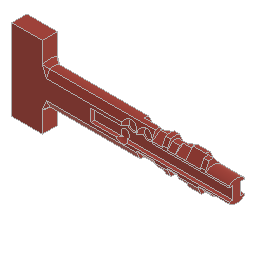
Protec (cam compatible) (Autodesk Fusion 360 design; units mm, degrees)
Autodesk Fusion 360 part; units mm, degrees
note: some values were not read from the file. Chosen so that the rebuilt part matches the saved one: which pieces of a blend or face edit are solid.
sketch "profile" plane through (0, 0, 0) normal (1, 0, 0) x (0, 1, 0)
  line L0 (0, 0) -> (3.3, 0) construction
  line L1 (3.3, 0) -> (3.3, 3.3) construction
  line L2 (3.3, 3.3) -> (4.05, 3.3) construction
  line L3 (3.3, 3.3) -> (2.55, 3.3) construction
  line L4 (4.05, 3.3) -> (4.05, 4.5)
  line L5 (4.05, 3.3) -> (4.05, 2.1)
  line L6 (2.55, 3.3) -> (2.55, 4.5)
  line L7 (2.55, 3.3) -> (2.55, 2.1)
  line L8 (4.05, 4.5) -> (4.775, 4.5)
  line L9 (4.05, 2.1) -> (4.775, 2.1)
  line L10 (2.55, 2.1) -> (1.825, 2.1)
  line L11 (2.55, 4.5) -> (1.825, 4.5)
  line L12 (4.775, 4.5) -> (4.775, 5.165)
  line L13 (4.775, 2.1) -> (4.775, 1.435)
  line L14 (1.825, 2.1) -> (1.825, 1.435)
  line L15 (1.825, 4.5) -> (1.825, 5.165)
  line L16 (4.775, 5.165) -> (4.1589, 6.4863)
  line L17 (4.775, 5.165) -> (1.825, 5.165) construction
  line L18 (1.825, 1.435) -> (2.4411, 0.1137)
  line L19 (1.825, 5.165) -> (2.4411, 6.4863)
  line L20 (1.825, 5.165) -> (4.775, 5.165) construction
  line L21 (4.775, 1.435) -> (4.1589, 0.1137)
  arc A0 (4.1589, 6.4863) -> (2.4411, 6.4863) centre (3.3, 3.3) ccw
  arc A1 (2.4411, 0.1137) -> (4.1589, 0.1137) centre (3.3, 3.3) ccw
  dimension "d1" = 3.3
  dimension "d2" = 3.3
  dimension "d3" = 0.75
  dimension "d4" = 1.2
  dimension "d5" = 0.725
  dimension "d6" = 65
  dimension "d7" = 65
  dimension "d8" = 3.3
  dimension "d9" = 4.25
  constraint coincident L0.start origin
  constraint horizontal L0
  constraint perpendicular L0 L1
  constraint perpendicular L1 L2
  constraint perpendicular L1 L3
  constraint equal L2 L3
  constraint perpendicular L2 L4
  constraint perpendicular L2 L5
  constraint perpendicular L3 L6
  constraint perpendicular L3 L7
  constraint perpendicular L4 L8
  constraint perpendicular L5 L9
  constraint perpendicular L7 L10
  constraint perpendicular L6 L11
  constraint equal L6 L7
  constraint equal L5 L7
  constraint equal L4 L5
  constraint equal L8 L9
  constraint equal L9 L10
  constraint equal L10 L11
  constraint perpendicular L8 L12
  constraint perpendicular L9 L13
  constraint perpendicular L10 L14
  constraint perpendicular L11 L15
  constraint equal L12 L15
  constraint equal L14 L15
  constraint equal L13 L14
  constraint horizontal L17
  constraint parallel L16 L18
  constraint horizontal L20
  constraint equal L16 L19
  constraint parallel L19 L21
  constraint equal L18 L21
  constraint equal L16 L18
  constraint coincident L1.end L2.start
  measures "d1" distance of L0.start L0.end
  measures "d2" distance of L0.end L1.end
  measures "d3" distance of L1.end L2.end
  measures "d4" distance of L2.end L4.end
  measures "d5" distance of L4.end L8.end
  measures "d6" angle of L16 L17
  measures "d7" angle of L19 L20
  measures "d8" radius of A0
  measures "d9" distance of L16 L18
extrude "Extrude1" add sketch "profile" against normal blind 42.57 makes body 1
ref_plane "WorkPlane1" through (-21.285, 3.3, 3.3) normal (0, -1, 0) x (0, 0, 1)
sketch "bow" plane through (-42.57, 0, 0) normal (-1, 0, 0) x (0, -1, 0)
  line L0 (-2.55, 2.1) -> (-2.55, 4.5)
  line L1 (-2.55, 4.5) -> (-1.825, 4.5)
  line L2 (-1.825, 4.5) -> (-1.825, 5.165)
  line L3 (-1.825, 5.165) -> (-2.4411, 6.4863)
  arc A0 (-2.4411, 6.4863) -> (-4.1589, 6.4863) centre (-3.3, 3.3) ccw
  line L4 (-4.1589, 6.4863) -> (-4.775, 5.165)
  line L5 (-4.775, 5.165) -> (-4.775, 4.5)
  line L6 (-4.775, 4.5) -> (-4.05, 4.5)
  line L7 (-4.05, 4.5) -> (-4.05, 2.1)
  line L8 (-4.05, 2.1) -> (-4.775, 2.1)
  line L9 (-4.775, 2.1) -> (-4.775, 1.435)
  line L10 (-4.775, 1.435) -> (-4.1589, 0.1137)
  arc A1 (-4.1589, 0.1137) -> (-2.4411, 0.1137) centre (-3.3, 3.3) ccw
  line L11 (-2.4411, 0.1137) -> (-1.825, 1.435)
  line L12 (-1.825, 1.435) -> (-1.825, 2.1)
  line L13 (-1.825, 2.1) -> (-2.55, 2.1)
  circle A2 centre (-3.3, 3.3) radius 3.3 construction
  line L14 (-1.825, 5.165) -> (-1.825, 6.252)
  line L15 (-4.775, 5.165) -> (-4.775, 6.252)
  line L16 (-1.825, 1.435) -> (-1.825, 0.348)
  line L17 (-4.775, 1.435) -> (-4.775, 0.348)
  line L18 (-1.825, 6.252) -> (-1.825, 11.252)
  line L19 (-4.775, 6.252) -> (-4.775, 11.252)
  line L20 (-1.825, 0.348) -> (-1.825, -4.652)
  line L21 (-4.775, 0.348) -> (-4.775, -4.652)
  line L22 (-1.825, 11.252) -> (-4.775, 11.252)
  line L23 (-4.775, -4.652) -> (-1.825, -4.652)
  line L24 (-1.825, 1.435) -> (-1.825, 5.165)
  line L25 (-4.775, 5.165) -> (-4.775, 1.435)
  point P0 (-1.825, 5.165)
  point P1 (-4.775, 5.165)
  point P2 (-4.775, 1.435)
  point P3 (-1.825, 1.435)
  dimension "d12" = 6.6
  dimension "d13" = 5
  constraint concentric A0 A2
  constraint coincident P0 L2.end
  constraint coincident A2 L14.end
  constraint parallel L2 L14
  constraint coincident P1 L4.end
  constraint coincident A2 L15.end
  constraint parallel L5 L15
  constraint coincident P3 L11.end
  constraint coincident A2 L16.end
  constraint parallel L12 L16
  constraint coincident P2 L9.end
  constraint coincident A2 L17.end
  constraint parallel L9 L17
  constraint parallel L14 L18
  constraint parallel L15 L19
  constraint parallel L16 L20
  constraint parallel L17 L21
  constraint equal L20 L21
  constraint equal L19 L21
  constraint equal L18 L19
  measures "d12" diameter of A2
  measures "d13" distance of L14.end L18.end
sketch "dss holes + dc align" plane through (0, 3.3, 0) normal (0, -1, 0) x (-1, 0, 0)
  line L0 (0, 0) -> (0, -3.3) construction
  line L1 (0, -3.3) -> (19.57, -3.3) construction
  line L2 (19.57, -3.3) -> (21.07, -3.3) construction
  line L3 (21.07, -3.3) -> (21.07, -4.1) construction
  line L4 (21.07, -3.3) -> (21.07, -2.5) construction
  line L5 (19.57, -3.3) -> (19.57, -4.9) construction
  line L6 (19.57, -3.3) -> (19.57, -1.7) construction
  circle A0 centre (19.57, -4.9) radius 0.9
  circle A1 centre (19.57, -1.7) radius 0.9
  circle A2 centre (16.57, -4.9) radius 0.9
  circle A3 centre (16.57, -1.7) radius 0.9
  point P0 (21.07, -4.1)
  point P1 (21.07, -2.5)
  dimension "d14" = 3.3
  dimension "d15" = 19.57
  dimension "d16" = 1.5
  dimension "d17" = 0.8
  dimension "d18" = 1.6
  dimension "d19" = 1.8
  dimension "d20" = 3
  dimension "d21" = 1.6
  dimension "d22" = 3
  dimension "d23" = 1.6
  constraint coincident L0.start origin
  constraint vertical L0
  constraint perpendicular L0 L1
  constraint parallel L1 L2
  constraint perpendicular L2 L3
  constraint perpendicular L2 L4
  constraint equal L3 L4
  constraint perpendicular L2 L5
  constraint perpendicular L2 L6
  constraint equal L5 L6
  constraint coincident L5.end A0.centre
  constraint coincident L6.end A1.centre
  constraint equal A0 A1
  constraint equal A0 A2
  constraint equal A0 A3
  constraint coincident P0 L3.end
  constraint coincident P1 L4.end
  measures "d14" distance of L0.start L0.end
  measures "d15" distance of L0.end L1.end
  measures "d16" distance of L1.end L2.end
  measures "d17" distance of L2.end P0
  measures "d18" distance of L1.end L5.end
  measures "d19" diameter of A0
  measures "d20" distance of L5.end A2.centre
  measures "d21" distance of L1 A2.centre
  measures "d22" distance of L6.end A3.centre
  measures "d23" distance of L1 A3.centre
sketch "dc bearings" plane through (0, 0, 0) normal (1, 0, 0) x (0, 1, 0)
  line L0 (0, 0) -> (3.3, 0) construction
  line L1 (3.3, 0) -> (3.3, 3.3) construction
  line L2 (3.3, 3.3) -> (1.4542, 2.8398) construction
  line L3 (3.3, 3.3) -> (2.3, 3.3) construction
  line L4 (3.3, 3.3) -> (5.1458, 3.7602) construction
  circle A0 centre (1.4542, 2.8398) radius 1.375
  circle A1 centre (5.1458, 3.7602) radius 1.375
  point P0 (1.4542, 2.8398)
  point P1 (5.1458, 3.7602)
  dimension "d24" = 3.3
  dimension "d25" = 3.3
  dimension "d26" = 14
  dimension "d27" = 1.9023
  dimension "d28" = 1
  dimension "d29" = 2.75
  constraint coincident L0.start origin
  constraint horizontal L0
  constraint perpendicular L0 L1
  constraint horizontal L3
  constraint parallel L2 L4
  constraint equal L2 L4
  constraint coincident P0 L2.end
  constraint coincident P1 L4.end
  constraint equal A0 A1
  measures "d24" distance of L0.start L0.end
  measures "d25" distance of L0.end L1.end
  measures "d26" angle of L2 L3
  measures "d27" distance of L1.end P0
  measures "d28" distance of L1.end L3.end
  measures "d29" diameter of A0
extrude "bow (1)" add sketch "bow" against normal blind 6 bodies 1
extrude "shaft strength" add 2 faces at (-36.57, 2.3083, 2.9) (-36.57, 4.5333, 3.7) along direction (1, 0, 0) blind 9.5 on bodies 1 bodies 1
chamfer "Chamfer1" distance 0.8 angle 45 6 edges at (-36.57, 2.1331, 5.8256) (-36.57, 3.3, 6.6) (-36.57, 2.1331, 0.7744) (-36.57, 4.4669, 5.8256) (-36.57, 3.3, 0) (-36.57, 4.4669, 0.7744) on bodies 1
extrude "dc bearings (1)" add sketch "dc bearings" along normal mid plane 2.75 separate body makes body 2 at (0.9167, 6.5191, 3.6917) makes body 3 at (0.9167, 2.8275, 2.7712)
fillet "Fillet1" radius 1.375 4 edges at (-1.375, 3.8639, 4.2574) (1.375, 3.8639, 3.263) (-1.375, 0.1722, 3.337) (1.375, 0.1722, 2.3426) on bodies 2 3
move_body "Move1" bodies 2 3 to x (1, 0, 0) y (0, 1, 0) z (0, 0, 1) at (-21.07, 0, 0)
extrude "Extrude5" cut sketch "dss holes + dc align" along normal blind 0.9 draft 35 from surface at 0.575 contours A0 | A2 bodies 1
extrude "Extrude6" cut sketch "dss holes + dc align" against normal blind 0.9 draft 35 from surface at -0.575 contours A1 | A3 bodies 1
combine "Combine1" operation cut target body 1 tool bodies 2 3
sketch "1 cut" plane through (0, 0, 0) normal (1, 0, 0) x (0, 1, 0)
  line L0 (0, 0) -> (3.3, 0) construction
  line L1 (3.3, 0) -> (3.3, 3.3) construction
  line L2 (3.3, 3.3) -> (4.05, 3.3) construction
  line L3 (4.05, 3.3) -> (4.05, 4.5)
  line L4 (4.05, 4.5) -> (4.775, 4.5)
  line L5 (4.05, 3.3) -> (4.05, 2.1)
  line L6 (4.05, 2.1) -> (4.775, 2.1)
  line L7 (2.55, 2.1) -> (1.825, 2.1)
  line L8 (2.55, 3.3) -> (2.55, 2.1)
  line L9 (2.55, 3.3) -> (2.55, 4.5)
  line L10 (2.55, 4.5) -> (1.825, 4.5)
  line L11 (4.775, 4.5) -> (4.775, 4.8481)
  line L12 (1.825, 2.1) -> (1.825, 1.7519)
  line L13 (1.825, 4.5) -> (1.825, 5.165)
  line L14 (4.775, 2.1) -> (4.775, 1.435)
  circle A0 centre (3.3, 3.3) radius 3.3 construction
  line L15 (4.775, 4.8481) -> (3.305, 6.6)
  line L16 (4.775, 4.8481) -> (1.825, 4.8481) construction
  line L17 (1.825, 1.7519) -> (3.295, 0)
  line L18 (1.825, 5.165) -> (2.4411, 6.4863)
  line L19 (1.825, 5.165) -> (4.509, 5.165) construction
  line L20 (4.775, 1.435) -> (4.1589, 0.1137)
  arc A1 (3.305, 6.6) -> (2.4411, 6.4863) centre (3.3, 3.3) ccw
  arc A2 (3.295, 0) -> (4.1589, 0.1137) centre (3.3, 3.3) ccw
  circle A3 centre (3.3, 3.3) radius 4.125
  dimension "d48" = 3.3
  dimension "d49" = 3.3
  dimension "d50" = 0.75
  dimension "d51" = 1.2
  dimension "d52" = 0.725
  dimension "d53" = 6.6
  dimension "d54" = 50
  dimension "d55" = 4.25
  dimension "d56" = 65
  dimension "d57" = 4.25
  dimension "d58" = 3.3
  dimension "d59" = 3.3
  dimension "d60" = 8.25
  constraint coincident L0.start origin
  constraint horizontal L0
  constraint perpendicular L0 L1
  constraint perpendicular L1 L2
  constraint perpendicular L2 L3
  constraint perpendicular L3 L4
  constraint perpendicular L2 L5
  constraint perpendicular L5 L6
  constraint equal L3 L5
  constraint equal L4 L6
  constraint symmetric L1 L2.end L8.start
  constraint symmetric L1 L3.end L9.end
  constraint symmetric L1 L4.end L10.end
  constraint symmetric L1 L5.end L7.start
  constraint symmetric L1 L6.end L7.end
  constraint perpendicular L4 L11
  constraint perpendicular L7 L12
  constraint equal L11 L12
  constraint perpendicular L10 L13
  constraint perpendicular L6 L14
  constraint equal L13 L14
  constraint coincident L1.end L2.start
  constraint horizontal L16
  constraint coincident A0 L15.end
  constraint coincident A0 L17.end
  constraint parallel L15 L17
  constraint horizontal L19
  constraint coincident A0 L18.end
  constraint coincident A0 L20.end
  constraint parallel L18 L20
  constraint coincident L13 L16.end
  constraint coincident L15 L19.end
  constraint concentric A2 A3
  measures "d48" distance of L0.start L0.end
  measures "d49" distance of L0.end L1.end
  measures "d50" distance of L1.end L2.end
  measures "d51" distance of L2.end L3.end
  measures "d52" distance of L3.end L4.end
  measures "d53" diameter of A0
  measures "d54" angle of L15 L16
  measures "d55" distance of L15 L17
  measures "d56" angle of L18 L19
  measures "d57" distance of L18 L20
  measures "d58" radius of A1
  measures "d59" radius of A2
  measures "d60" diameter of A3
sketch "2 cut" plane through (0, 0, 0) normal (1, 0, 0) x (0, 1, 0)
  line L0 (1.825, 5.165) -> (2.4411, 6.4863) construction
  line L1 (1.825, 4.5) -> (1.825, 5.165) construction
  line L2 (2.55, 4.5) -> (1.825, 4.5) construction
  line L3 (2.55, 3.3) -> (2.55, 4.5) construction
  line L4 (2.55, 3.3) -> (2.55, 2.1) construction
  line L5 (2.55, 2.1) -> (1.825, 2.1) construction
  line L6 (1.825, 2.1) -> (1.825, 1.7519) construction
  line L7 (1.825, 1.7519) -> (3.295, 0) construction
  arc A0 (3.295, 0) -> (4.1589, 0.1137) centre (3.3, 3.3) ccw construction
  line L8 (4.775, 1.435) -> (4.1589, 0.1137) construction
  line L9 (4.775, 2.1) -> (4.775, 1.435) construction
  line L10 (4.05, 2.1) -> (4.775, 2.1) construction
  line L11 (4.05, 3.3) -> (4.05, 2.1) construction
  line L12 (4.05, 3.3) -> (4.05, 4.5) construction
  line L13 (4.05, 4.5) -> (4.775, 4.5) construction
  line L14 (4.775, 4.5) -> (4.775, 4.8481) construction
  arc A1 (3.305, 6.6) -> (2.4411, 6.4863) centre (3.3, 3.3) ccw construction
  line L15 (4.775, 4.8481) -> (3.305, 6.6) construction
  circle A2 centre (3.3, 3.3) radius 4.125 construction
  line L16 (3.3, 3.3) -> (3.3, 4.3) construction
  line L17 (4.775, 5.165) -> (4.1589, 6.4863)
  line L18 (4.775, 4.5) -> (4.775, 5.165)
  line L19 (4.05, 4.5) -> (4.775, 4.5)
  line L20 (4.05, 3.3) -> (4.05, 4.5)
  line L21 (4.05, 3.3) -> (4.05, 2.1)
  line L22 (4.05, 2.1) -> (4.775, 2.1)
  line L23 (4.775, 2.1) -> (4.775, 1.7519)
  line L24 (4.775, 1.7519) -> (3.305, 0)
  arc A3 (2.4411, 0.1137) -> (3.305, 0) centre (3.3, 3.3) ccw
  line L25 (1.825, 1.435) -> (2.4411, 0.1137)
  line L26 (1.825, 2.1) -> (1.825, 1.435)
  line L27 (2.55, 2.1) -> (1.825, 2.1)
  line L28 (2.55, 3.3) -> (2.55, 2.1)
  line L29 (2.55, 3.3) -> (2.55, 4.5)
  line L30 (2.55, 4.5) -> (1.825, 4.5)
  line L31 (1.825, 4.5) -> (1.825, 4.8481)
  arc A4 (4.1589, 6.4863) -> (3.295, 6.6) centre (3.3, 3.3) ccw
  line L32 (1.825, 4.8481) -> (3.295, 6.6)
  circle A5 centre (3.3, 3.3) radius 4.125
  dimension "d61" = 1
  constraint coincident A0.centre A1.centre
  constraint parallel L3 L16
  constraint symmetric L0.start L16 L17.start
  constraint symmetric L0.end L16 L17.end
  constraint symmetric L1.start L16 L13.end
  constraint symmetric L2.start L16 L12.end
  constraint symmetric L3.start L16 L11.start
  constraint symmetric L4.end L16 L10.start
  constraint symmetric L5.end L16 L9.start
  constraint symmetric L6.end L16 L23.end
  constraint symmetric L7.end L16 L24.end
  constraint symmetric A0.end L16 A3.start
  constraint symmetric A0 L16 A3
  constraint symmetric L8.start L16 L25.start
  constraint symmetric L9.start L16 L5.end
  constraint symmetric L10.start L16 L4.end
  constraint symmetric L11.start L16 L3.start
  constraint symmetric L12.end L16 L2.start
  constraint symmetric L13.end L16 L1.start
  constraint symmetric L14.end L16 L31.end
  constraint symmetric A1.start L16 A4.end
  constraint symmetric A1 L16 A4
  constraint symmetric A2 L16 A5
  measures "d61" distance of A0.centre L16.end
sketch "3 cut" plane through (0, 0, 0) normal (1, 0, 0) x (0, 1, 0)
  line L0 (0, 0) -> (3.3, 0) construction
  line L1 (3.3, 0) -> (3.3, 3.3) construction
  line L2 (3.3, 3.3) -> (4.05, 3.3) construction
  line L3 (2.55, 3.3) -> (2.55, 2.1)
  line L4 (2.55, 2.1) -> (1.825, 2.1)
  line L5 (2.55, 3.3) -> (2.55, 4.5)
  line L6 (2.55, 4.5) -> (1.825, 4.5)
  line L7 (4.05, 4.5) -> (4.775, 4.5)
  line L8 (4.05, 3.3) -> (4.05, 4.5)
  line L9 (4.05, 3.3) -> (4.05, 2.1)
  line L10 (4.05, 2.1) -> (4.775, 2.1)
  line L11 (4.775, 4.5) -> (4.775, 4.8613)
  line L12 (1.825, 2.1) -> (1.825, 1.7387)
  line L13 (1.825, 4.5) -> (1.825, 5.165)
  line L14 (4.775, 2.1) -> (4.775, 1.435)
  circle A0 centre (3.3, 3.3) radius 2.7 construction
  line L15 (4.775, 4.8613) -> (3.1544, 5.9961)
  line L16 (4.775, 4.8613) -> (1.825, 4.8613) construction
  line L17 (1.825, 1.7387) -> (3.4456, 0.6039)
  line L18 (1.825, 5.165) -> (2.078, 5.7077)
  line L19 (1.825, 5.165) -> (4.3413, 5.165) construction
  line L20 (4.775, 1.435) -> (4.522, 0.8923)
  arc A1 (3.1544, 5.9961) -> (2.078, 5.7077) centre (3.3, 3.3) ccw
  arc A2 (3.4456, 0.6039) -> (4.522, 0.8923) centre (3.3, 3.3) ccw
  circle A3 centre (3.3, 3.3) radius 4.125
  dimension "d62" = 3.3
  dimension "d63" = 3.3
  dimension "d64" = 0.75
  dimension "d65" = 5.4
  dimension "d66" = 35
  dimension "d67" = 4.25
  dimension "d68" = 65
  dimension "d69" = 4.25
  dimension "d70" = 2.7
  dimension "d71" = 2.7
  dimension "d72" = 8.25
  constraint coincident L0.start origin
  constraint horizontal L0
  constraint perpendicular L0 L1
  constraint perpendicular L1 L2
  constraint coincident L7.end L11.start
  constraint perpendicular L7 L11
  constraint coincident L4.end L12.start
  constraint perpendicular L4 L12
  constraint equal L11 L12
  constraint coincident L6.end L13.start
  constraint perpendicular L6 L13
  constraint coincident L10.end L14.start
  constraint perpendicular L10 L14
  constraint equal L13 L14
  constraint coincident L1.end L2.start
  constraint horizontal L16
  constraint coincident A0 L15.end
  constraint coincident A0 L17.end
  constraint parallel L15 L17
  constraint horizontal L19
  constraint coincident A0 L18.end
  constraint coincident A0 L20.end
  constraint parallel L18 L20
  constraint concentric A2 A3
  constraint coincident L13 L16.end
  constraint coincident L15 L19.end
  measures "d62" distance of L0.start L0.end
  measures "d63" distance of L0.end L1.end
  measures "d64" distance of L1.end L2.end
  measures "d65" diameter of A0
  measures "d66" angle of L15 L16
  measures "d67" distance of L15 L17
  measures "d68" angle of L18 L19
  measures "d69" distance of L18 L20
  measures "d70" radius of A2
  measures "d71" radius of A1
  measures "d72" diameter of A3
sketch "4 cut" plane through (0, 0, 0) normal (1, 0, 0) x (0, 1, 0)
  line L0 (0, 0) -> (3.3, 0) construction
  line L1 (3.3, 0) -> (3.3, 3.3) construction
  line L2 (3.3, 3.3) -> (4.05, 3.3) construction
  line L3 (2.55, 4.5) -> (1.825, 4.5)
  line L4 (2.55, 3.3) -> (2.55, 4.5)
  line L5 (2.55, 3.3) -> (2.55, 2.1)
  line L6 (2.55, 2.1) -> (1.825, 2.1)
  line L7 (4.05, 2.1) -> (4.775, 2.1)
  line L8 (4.05, 3.3) -> (4.05, 2.1)
  line L9 (4.05, 3.3) -> (4.05, 4.5)
  line L10 (4.05, 4.5) -> (4.775, 4.5)
  line L11 (4.775, 4.5) -> (4.775, 4.8481)
  line L12 (1.825, 2.1) -> (1.825, 1.7519)
  line L13 (4.775, 2.1) -> (4.775, 1.7519)
  line L14 (1.825, 4.5) -> (1.825, 4.8481)
  circle A0 centre (3.3, 3.3) radius 2.7 construction
  line L15 (4.775, 4.8481) -> (3.8572, 5.9419)
  line L16 (4.775, 4.8481) -> (1.825, 4.8481) construction
  line L17 (1.825, 1.7519) -> (2.7428, 0.6581)
  line L18 (1.825, 4.8481) -> (2.7428, 5.9419)
  line L19 (1.825, 4.8481) -> (4.775, 4.8481) construction
  line L20 (4.775, 1.7519) -> (3.8572, 0.6581)
  arc A1 (3.8572, 5.9419) -> (2.7428, 5.9419) centre (3.3, 3.3) ccw
  arc A2 (2.7428, 0.6581) -> (3.8572, 0.6581) centre (3.3, 3.3) ccw
  circle A3 centre (3.3, 3.3) radius 4.125
  dimension "d73" = 3.3
  dimension "d74" = 3.3
  dimension "d75" = 0.75
  dimension "d76" = 5.4
  dimension "d77" = 50
  dimension "d78" = 4.25
  dimension "d79" = 50
  dimension "d80" = 8.25
  constraint coincident L0.start origin
  constraint horizontal L0
  constraint perpendicular L0 L1
  constraint perpendicular L1 L2
  constraint coincident L10.end L11.start
  constraint perpendicular L10 L11
  constraint coincident L6.end L12.start
  constraint perpendicular L6 L12
  constraint coincident L7.end L13.start
  constraint perpendicular L7 L13
  constraint coincident L3.end L14.start
  constraint perpendicular L3 L14
  constraint equal L12 L13
  constraint equal L12 L14
  constraint equal L11 L14
  constraint coincident L1.end L2.start
  constraint horizontal L16
  constraint coincident A0 L15.end
  constraint coincident A0 L17.end
  constraint parallel L15 L17
  constraint horizontal L19
  constraint coincident A0 L18.end
  constraint coincident A0 L20.end
  constraint parallel L18 L20
  constraint concentric A0 A3
  measures "d73" distance of L0.start L0.end
  measures "d74" distance of L0.end L1.end
  measures "d75" distance of L1.end L2.end
  measures "d76" diameter of A0
  measures "d77" angle of L15 L16
  measures "d78" distance of L15 L17
  measures "d79" angle of L18 L19
  measures "d80" diameter of A3
sketch "5 cut" plane through (0, 0, 0) normal (1, 0, 0) x (0, 1, 0)
  circle A0 centre (3.3, 3.3) radius 4.125 construction
  line L0 (1.825, 2.1) -> (1.825, 1.7387) construction
  line L1 (1.825, 1.7387) -> (3.4456, 0.6039) construction
  arc A1 (3.4456, 0.6039) -> (4.522, 0.8923) centre (3.3, 3.3) ccw construction
  line L2 (4.775, 1.435) -> (4.522, 0.8923) construction
  line L3 (4.775, 2.1) -> (4.775, 1.435) construction
  line L4 (4.05, 2.1) -> (4.775, 2.1) construction
  line L5 (4.05, 3.3) -> (4.05, 2.1) construction
  line L6 (2.55, 2.1) -> (1.825, 2.1) construction
  line L7 (2.55, 3.3) -> (2.55, 2.1) construction
  line L8 (4.05, 3.3) -> (4.05, 4.5) construction
  line L9 (2.55, 3.3) -> (2.55, 4.5) construction
  line L10 (2.55, 4.5) -> (1.825, 4.5) construction
  line L11 (1.825, 4.5) -> (1.825, 5.165) construction
  line L12 (1.825, 5.165) -> (2.078, 5.7077) construction
  arc A2 (3.1544, 5.9961) -> (2.078, 5.7077) centre (3.3, 3.3) ccw construction
  line L13 (4.775, 4.8613) -> (3.1544, 5.9961) construction
  line L14 (4.775, 4.5) -> (4.775, 4.8613) construction
  line L15 (4.05, 4.5) -> (4.775, 4.5) construction
  line L16 (3.3, 3.3) -> (3.3, 4.3) construction
  line L17 (1.825, 4.5) -> (1.825, 4.8613)
  arc A3 (4.522, 5.7077) -> (3.4456, 5.9961) centre (3.3, 3.3) ccw
  line L18 (4.775, 5.165) -> (4.522, 5.7077)
  line L19 (4.775, 4.5) -> (4.775, 5.165)
  line L20 (1.825, 4.8613) -> (3.4456, 5.9961)
  line L21 (2.55, 2.1) -> (1.825, 2.1)
  line L22 (2.55, 3.3) -> (2.55, 2.1)
  line L23 (2.55, 3.3) -> (2.55, 4.5)
  line L24 (2.55, 4.5) -> (1.825, 4.5)
  line L25 (4.05, 2.1) -> (4.775, 2.1)
  line L26 (4.05, 3.3) -> (4.05, 2.1)
  line L27 (4.05, 4.5) -> (4.775, 4.5)
  line L28 (4.05, 3.3) -> (4.05, 4.5)
  line L29 (4.775, 2.1) -> (4.775, 1.7387)
  arc A4 (2.078, 0.8923) -> (3.1544, 0.6039) centre (3.3, 3.3) ccw
  line L30 (1.825, 1.435) -> (2.078, 0.8923)
  line L31 (1.825, 2.1) -> (1.825, 1.435)
  line L32 (4.775, 1.7387) -> (3.1544, 0.6039)
  circle A5 centre (3.3, 3.3) radius 4.125
  dimension "d81" = 1
  constraint coincident A0.centre A1.centre
  constraint perpendicular L10 L16
  constraint symmetric A0 L16 A5
  constraint symmetric L0.start L16 L3.start
  constraint symmetric L0.end L16 L29.end
  constraint symmetric L1.end L16 A4.end
  constraint symmetric A1.end L16 A4.start
  constraint symmetric A1 L16 A4
  constraint symmetric L2.start L16 L30.start
  constraint symmetric L3.start L16 L0.start
  constraint symmetric L4.start L16 L6.start
  constraint symmetric L5.start L16 L7.start
  constraint symmetric L6.start L16 L4.start
  constraint symmetric L7.start L16 L5.start
  constraint symmetric L8.end L16 L9.end
  constraint symmetric L9.end L16 L8.end
  constraint symmetric L10.end L16 L14.start
  constraint symmetric L11.end L16 L18.start
  constraint symmetric L12.end L16 A3.start
  constraint symmetric A2.start L16 A3.end
  constraint symmetric A2 L16 A3
  constraint symmetric L13.start L16 L17.end
  constraint symmetric L14.start L16 L10.end
  measures "d81" distance of A0.centre L16.end
sketch "6 cut" plane through (0, 0, 0) normal (1, 0, 0) x (0, 1, 0)
  line L0 (0, 0) -> (3.3, 0) construction
  line L1 (3.3, 0) -> (3.3, 3.3) construction
  line L2 (4.775, 4.8613) -> (3.1544, 5.9961) construction
  circle A0 centre (3.3, 3.3) radius 2.125
  circle A1 centre (3.3, 3.3) radius 4.125
  dimension "d82" = 3.3
  dimension "d83" = 3.3
  dimension "d84" = 8.25
  constraint coincident L0.start origin
  constraint horizontal L0
  constraint perpendicular L0 L1
  constraint coincident L1.end A0.centre
  constraint tangent L2 A0
  constraint concentric A0 A1
  measures "d82" distance of L0.start L0.end
  measures "d83" distance of L0.end L1.end
  measures "d84" diameter of A1
extrude "tip" cut sketch "6 cut" against normal blind 3.07 bodies 1
extrude "1" cut sketch "6 cut" along normal mid plane 2 from surface at -3.57 bodies 1
extrude "2" cut sketch "1 cut" along normal mid plane 2 from surface at -5.07 bodies 1
extrude "3" cut sketch "2 cut" along normal mid plane 2 from surface at -6.57 bodies 1
extrude "4" cut sketch "2 cut" along normal mid plane 2 from surface at -8.07 bodies 1
extrude "5" cut sketch "5 cut" along normal mid plane 2 from surface at -9.57 bodies 1
extrude "6" cut sketch "4 cut" along normal mid plane 2 from surface at -11.07 bodies 1
extrude "8" cut sketch "5 cut" along normal mid plane 2 from surface at -14.07 bodies 1
extrude "9" cut sketch "1 cut" along normal mid plane 2 from surface at -15.57 bodies 1
extrude "10" cut sketch "1 cut" along normal mid plane 2 from surface at -17.07 bodies 1
equation "d2 = d1"
equation "d3 = ( 1.5 / 2 ) * 1 mm"
equation "d4 = ( 2.4 / 2 ) * 1 mm"
equation "d5 = ( 2.95 / 2 ) * 1 mm - d3"
equation "d6 = 90 deg - 25 deg"
equation "d7 = d6"
equation "d10 = -( 2.57 mm + 35 mm + 2 mm + 3 mm )"
equation "d12 = d1 * 2"
equation "d14 = d1"
equation "d15 = 19.17 mm + 0.4 mm"
equation "d21 = d18"
equation "d22 = d20"
equation "d23 = d18"
equation "d24 = d1"
equation "d25 = d1"
equation "d32 = 12.50 mm - 3 mm"
equation "d35 = ( 0.5 * 2.75 ) * 1 mm"
equation "d38 = ( 0.5 * 2.75 ) * 1 mm"
equation "d42 = 0.575 mm"
equation "d43 = 0.90 mm"
equation "d44 = 35 deg"
equation "d45 = -d42"
equation "d46 = -d43"
equation "d47 = d44"
equation "d48 = d1"
equation "d49 = d1"
equation "d50 = d3"
equation "d51 = d4"
equation "d52 = d5"
equation "d53 = d1 * 2"
equation "d54 = 65 deg - 15 deg"
equation "d57 = d55"
equation "d60 = d1 * 2.5"
equation "d62 = d1"
equation "d63 = d1"
equation "d64 = d3"
equation "d66 = 65 deg - 30 deg"
equation "d69 = d67"
equation "d72 = d1 * 2.5"
equation "d73 = d1"
equation "d74 = d1"
equation "d75 = d3"
equation "d79 = d77"
equation "d80 = d1 * 2.5"
equation "d82 = d1"
equation "d83 = d1"
equation "d84 = d1 * 2.5"
equation "d87 = -2.07 mm - ( 1.5 * 1 mm )"
equation "d90 = -2.07 mm - ( 1.5 * 2 mm )"
equation "d93 = -2.07 mm - ( 1.5 * 3 mm )"
equation "d96 = -2.07 mm - ( 1.5 * 4 mm )"
equation "d99 = -2.07 mm - ( 1.5 * 5 mm )"
equation "d102 = -2.07 mm - ( 1.5 * 6 mm )"
equation "d105 = -2.07 mm - ( 1.5 * 8 mm )"
equation "d108 = -2.07 mm - ( 1.5 * 9 mm )"
equation "d111 = -2.07 mm - ( 1.5 * 10 mm )"
